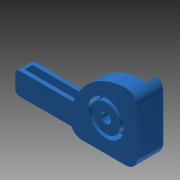
# Autodesk Inventor part: BedClipUltiBot
Saved by Autodesk Inventor 2015 SP1 (Build 190203100, 203)
## iProperties
Category: Print
Created: 2013-12-28
Part Number: BedClipUltiBot
Material: ABS Plastic
Document SubType Name: Modeling
Designer: Jack
Density: 1.06 g/cm^3
Appearance: Cyan
Mass: 6.75073 g
Surface Area: 45.8569 cm^2
Volume: 6.36862 cm^3
Catalog Web Link: N/A
Author: Jack
Title: Bed Clip Ultibots
Autodesk Inventor part; units mm, degrees
ref_plane "YZ Plane" through (0, 0, 0) normal (1, 0, 0) x (0, 1, 0)
ref_plane "XZ Plane" through (0, 0, 0) normal (0, 1, 0) x (-1, 0, 0)
ref_plane "XY Plane" through (0, 0, 0) normal (0, 0, 1) x (1, 0, 0)
sketch "Sketch1" plane through (0, 0, 0) normal (0, 1, 0) x (-1, 0, 0)
  arc A0 (-5, 0) -> (0, -5) centre (0, 0) ccw
  arc A1 (0.1667, 25.2972) -> (-5, 20.3) centre (0, 20.3) ccw
  line L0 (-5, 0) -> (-5, 20.3)
  arc A2 (23.8054, 8) -> (0.1667, 25.2972) centre (-0.7, -0.6883) ccw
  line L1 (48, -2) -> (24.5826, -2)
  arc A3 (20, -5) -> (24.5826, -2) centre (20, 0) ccw
  line L2 (0, -5) -> (20, -5)
  line L3 (50, 0) -> (50, 6)
  line L4 (48, 8) -> (23.8054, 8)
  arc A4 (50, 6) -> (48, 8) centre (48, 6) ccw
  arc A5 (48, -2) -> (50, 0) centre (48, 0) ccw
  point P0 (50, -2)
  point P1 (50, 8)
  dimension "d0" = 5
  dimension "d1" = 5
  dimension "d2" = 20.3
  dimension "d3" = 26
  dimension "d4" = 0.7
  dimension "d8" = 5
  dimension "d9" = 20
  dimension "d12" = 3
  dimension "d13" = 55
  dimension "d14" = 10
  dimension "d15" = 2
  constraints: 12 point on circle, 10 end point, 8 tangent, 6 centre point, 4 point on line, 2 perpendicular, 1 coincident, 1 equal radius, 1 horizontal alignment, 1 vertical, 1 vertical alignment
  measures "d0" radius of A0
  measures "d1" radius of A1
  measures "d2" distance of A1.centre point (0, 0)
  measures "d3" radius of A2
  measures "d4" horizontal distance of A2.centre point (0, 0)
  measures "d8" radius of A3
  measures "d9" distance of point (0, 0) A3.centre
  measures "d12" distance between parallel lines of L2 L1
  measures "d13" distance from line of L0 point (50, -2)
  measures "d14" distance of point (50, -2) point (50, 8)
  measures "d15" radius of A4
extrude "Extrusion1" add sketch "Sketch1" along normal blind 7
sketch "Sketch2" plane through (0, 7, 0) normal (0, 1, 0) x (1, 0, 0)
  arc A0 (5, 0) -> (0, 5) centre (0, 0) ccw projected
  line L0 (0, 5) -> (-20, 5) projected
  arc A1 (-0.1667, -25.2972) -> (5, -20.3) centre (0, -20.3) ccw projected
  line L1 (5, -20.3) -> (5, 0) projected
  line L2 (-24.5826, 2) -> (0, 2)
  arc A2 (2, 0) -> (0, 2) centre (0, 0) ccw
  line L3 (2, 0) -> (2, -24.8826)
  line L4 (-24.5826, 2) -> (-48, 2) projected
  arc A3 (-20, 5) -> (-24.5826, 2) centre (-20, 0) ccw projected
  line L5 (-50, 0) -> (-50, -6) projected
  arc A4 (-48, 2) -> (-50, 0) centre (-48, 0) ccw projected
  arc A5 (-50, -6) -> (-48, -8) centre (-48, -6) ccw projected
  line L6 (-48, -8) -> (-23.8054, -8) projected
  arc A6 (-23.8054, -8) -> (-0.1667, -25.2972) centre (0.7, 0.6883) ccw projected
  dimension "d16" = 3
  dimension "d17" = 3
  dimension "d18" = 2
  constraints: 4 end point, 4 point on circle, 1 centre point
  measures "d16" distance between parallel lines of L0 L2
  measures "d17" distance between parallel lines of L1 L3
  measures "d18" radius of A2
extrude "Extrusion2" add sketch "Sketch2" along normal blind 5.5 contours L1 A1 L3 A2 L2 A3 L0 A0
fillet "Fillet1" radius 1 8 edges at (3.5355, 12.5, -3.5355) (-10, 12.5, -5) (-22.7386, 12.5, -4.1833) (4.1833, 12.5, 23.0386) (5, 12.5, 10.15) (1.4142, 12.5, -1.4142) (2, 12.5, 12.4413) (-12.2913, 12.5, -2)
sketch "Sketch7" plane through (-24.5826, 0, -2) normal (0, 0, -1) x (-1, 0, 0)
  line L0 (0.4174, 1.75) -> (22.8174, 1.75)
  line L1 (22.8174, 1.75) -> (22.8174, 5.25)
  line L2 (22.8174, 5.25) -> (0.4174, 5.25)
  line L3 (0.4174, 5.25) -> (0.4174, 1.75)
  line L4 (25.4174, 0) -> (25.4174, 7) projected
  point P0 (23.4174, 7)
  point P1 (-24.5826, 0)
  dimension "d49" = 22.4
  dimension "d50" = 3.5
  dimension "d51" = 2.6
  dimension "d52" = 1.75
  constraints: 8 end point, 2 parallel, 1 horizontal, 1 perpendicular
  measures "d49" distance of L2.end L1.end
  measures "d50" distance of L1.end L0.end
  measures "d51" distance between parallel lines of L4 L1
  measures "d52" distance from line of point (23.417, 7) L2
extrude "Extrusion7" cut sketch "Sketch7" against normal up to next
sketch "Sketch8" plane through (0, 0, 0) normal (0, -1, 0) x (1, 0, 0)
  line L0 (5, 20.3) -> (5, 0) projected
  line L1 (0, -5) -> (-20, -5) projected
  circle A0 centre (-9, 9) radius 7.925
  circle A1 centre (-9, 9) radius 6.25
  dimension "d55" = 14
  dimension "d56" = 14
  dimension "d57" = 15.85
  dimension "d58" = 12.5
  constraints: 2 centre point, 1 coincident
  measures "d55" distance from line of L1 A0.centre
  measures "d56" distance from line of L0 A0.centre
  measures "d57" diameter of A0
  measures "d58" diameter of A1
extrude "Extrusion8" cut sketch "Sketch8" against normal blind 5
sketch "Sketch9" plane through (0, 7, 0) normal (0, 1, 0) x (1, 0, 0)
  circle A0 centre (-9, -9) radius 6.25 projected
hole "Hole1" at (-9, 7, 9) direction (0, -1, 0) diameter 4.5 end through all counterbore diameter 7.4 counterbore depth 4.5
body "Solid1"
